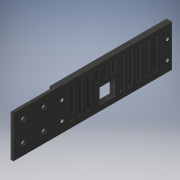
# Autodesk Inventor part: Base Left Front Panel
Saved by Autodesk Inventor 2019 (Build 230136000, 136)
## iProperties
Created: 2018-11-05
Part Number: Base Left Front Panel
Material: Generic
Document SubType Name: Modeling
Designer: Keith
Density: 1 g/cm^3
Appearance: Default
Author: Keith
## iProperties of the stored document Base Left Front Panel_3DPrint.ipt
Created: 2018-12-04
Part Number: Base Left Front Panel_3DPrint
Material: Generic
Document SubType Name: Modeling
Designer: Keith
Density: 1 g/cm^3
Appearance: Default
Author: Keith
Autodesk Inventor part; units mm, degrees
(part 1 of 2)
ref_plane "YZ Plane" through (0, 0, 0) normal (1, 0, 0) x (0, 1, 0)
sketch "Sketch1" plane through (0, 0, 0) normal (0, 1, 0) x (-1, 0, 0)
  line L0 (0, 0) -> (124, 0)
  line L1 (124, 0) -> (124, -124.7)
  line L2 (124, -124.7) -> (0, -124.7)
  line L3 (0, -124.7) -> (0, 0)
  line L4 (121.5, -2.5) -> (2.5, -2.5)
  line L5 (2.5, -2.5) -> (2.5, -122.2)
  line L6 (2.5, -122.2) -> (121.5, -122.2)
  line L7 (121.5, -122.2) -> (121.5, -2.5)
  line L8 (113, -2.5) -> (121.5, -2.5)
  line L9 (121.5, -2.5) -> (121.5, -11.25)
  line L10 (121.5, -11.25) -> (113, -11.25)
  line L11 (113, -11.25) -> (113, -2.5)
  line L12 (2.5, -11.25) -> (11, -11.25)
  line L13 (11, -11.25) -> (11, -2.5)
  line L14 (124, -124.7) -> (113, -124.7)
  line L15 (113, -124.7) -> (113, -112.7)
  line L16 (124, -112.7) -> (124, -124.7)
  line L17 (124, -112.7) -> (124, -104.2)
  line L18 (124, -104.2) -> (113, -104.2)
  line L19 (113, -104.2) -> (113, -112.7)
  line L20 (11, -124.7) -> (11, -112.7)
  line L21 (0, -104.2) -> (11, -104.2)
  line L22 (11, -104.2) -> (11, -112.7)
  line L23 (11, -11.25) -> (2.5, -11.25)
  line L24 (2.5, -11.25) -> (2.5, -2.5)
  line L25 (2.5, -2.5) -> (11, -2.5)
  line L26 (11, -2.5) -> (11, -11.25)
  line L27 (0, -104.2) -> (11, -104.2)
  line L28 (11, -104.2) -> (11, -124.7)
  line L29 (11, -124.7) -> (0, -124.7)
  line L30 (0, -124.7) -> (0, -104.2)
  dimension "d0" = 124
  dimension "d1" = 124.7
  dimension "d2" = 2.5
  dimension "d3" = 2.5
  dimension "d4" = 2.5
  dimension "d5" = 2.5
  dimension "d6" = 11.25
  dimension "d7" = 11
  dimension "d8" = 12
  dimension "d9" = 11
  dimension "d10" = 8.5
  dimension "d125" = 0
  dimension "d126" = 20.5
  constraints: 62 end point, 12 parallel, 6 horizontal, 6 perpendicular, 3 point on line
  measures "d0" distance of L1.end L2.end
  measures "d1" distance of L0.end L1.end
  measures "d2" distance between parallel lines of L1 L7
  measures "d3" distance between parallel lines of L0 L4
  measures "d4" distance between parallel lines of L3 L5
  measures "d5" distance between parallel lines of L2 L6
  measures "d6" distance between parallel lines of L0 L10
  measures "d7" distance between parallel lines of L1 L11
  measures "d8" distance of L14.end L15.end
  measures "d9" distance between parallel lines of L1 L15
  measures "d10" distance of L17.end L17.start
  measures "d125" distance between parallel lines of L2 L29
  measures "d126" distance between parallel lines of L2 L21
extrude "Extrusion1" add sketch "Sketch1" along normal blind 43 contours L0 L1 L18 L7 L4 L5 L21 L3 | L21 L5 L6 L20 L2 L3 | L1 L2 L15 L6 L7 L18 | L21 L22 L20 L6 L5 | L7 L6 L15 L19 L18 | L20 L6 L15 L2 | L5 L4 L13 L12 | L10 L11 L4 L7
sketch "Sketch2" plane through (0, 43, 0) normal (0, 1, 0) x (1, 0, 0)
  line L0 (-124, 124.7) -> (-124, 0) projected
  line L1 (-124, 0) -> (0, 0) projected
  line L2 (0, 0) -> (0, 124.7) projected
  line L3 (0, 124.7) -> (-124, 124.7) projected
  line L4 (-113, 122.2) -> (-113, 104.2) projected
  line L5 (-113, 122.2) -> (-11, 122.2) projected
  line L6 (-11, 104.2) -> (-11, 122.2) projected
  line L7 (-2.5, 104.2) -> (-11, 104.2) projected
  line L8 (-2.5, 104.2) -> (-2.5, 11.25) projected
  line L9 (-11, 11.25) -> (-2.5, 11.25) projected
  line L10 (-11, 2.5) -> (-11, 11.25) projected
  line L11 (-11, 2.5) -> (-113, 2.5) projected
  line L12 (-113, 2.5) -> (-113, 11.25) projected
  line L13 (-113, 11.25) -> (-121.5, 11.25) projected
  line L14 (-121.5, 11.25) -> (-121.5, 104.2) projected
  line L15 (-113, 104.2) -> (-121.5, 104.2) projected
  line L16 (-124, 124.7) -> (-124, 0) projected
  line L17 (0, 131.353) -> (-124, 131.353)
  line L18 (-124, 131.353) -> (-124, 119.353)
  line L19 (0, 119.353) -> (0, 131.353)
  line L20 (-11, 104.2) -> (-11, 122.2) projected
  line L21 (-113, 119.353) -> (-113, 122.2)
  line L22 (-113, 122.2) -> (-11, 122.2)
  line L23 (-11, 122.2) -> (-11, 119.353)
  line L24 (-124, 119.353) -> (-113, 119.353)
  line L25 (-11, 119.353) -> (0, 119.353)
  dimension "d13" = 12
  constraints: 16 end point, 3 equal length, 2 horizontal, 2 point on line, 1 perpendicular
  measures "d13" distance of L18.end L17.end
extrude "Extrusion2" cut sketch "Sketch2" against normal blind 11.4 contours L3 L2 L25 L6 L5 L4 L24 L0 | L18 L17 L19 L3
sketch "Sketch3" plane through (0, 31.6, 0) normal (0, 1, 0) x (1, 0, 0)
  line L0 (-124, 124.7) -> (0, 124.7) projected
  line L1 (-124, 124.7) -> (0, 124.7) projected
  line L2 (-124, 119.353) -> (-124, 124.7) projected
  line L3 (-113, 119.353) -> (-124, 119.353) projected
  line L4 (-113, 122.2) -> (-113, 119.353) projected
  line L5 (-11, 122.2) -> (-113, 122.2) projected
  line L6 (-11, 119.353) -> (-11, 122.2) projected
  line L7 (0, 119.353) -> (-11, 119.353) projected
  line L8 (0, 124.7) -> (0, 119.353) projected
  line L9 (-113, 122.2) -> (-11, 122.2)
  line L10 (-11, 122.2) -> (-11, 124.7)
  line L11 (-11, 124.7) -> (-113, 124.7)
  line L12 (-113, 124.7) -> (-113, 122.2)
  point P0 (0, 0)
  constraints: 8 end point, 2 parallel, 1 horizontal, 1 perpendicular, 1 point on line
extrude "Extrusion3" cut sketch "Sketch3" against normal through all contours L0 L10 L5 L12
sketch "Sketch4" plane through (0, 0, 0) normal (0, -1, 0) x (1, 0, 0)
  line L0 (-113, -104.2) -> (-113, -124.7) projected
  line L1 (-121.5, -104.2) -> (-113, -104.2) projected
  line L2 (-121.5, -104.2) -> (-121.5, -11.25) projected
  line L3 (-121.5, -11.25) -> (-113, -11.25) projected
  line L4 (-113, -11.25) -> (-113, -2.5) projected
  line L5 (-113, -2.5) -> (-11, -2.5) projected
  line L6 (-11, -11.25) -> (-11, -2.5) projected
  line L7 (-2.5, -11.25) -> (-11, -11.25) projected
  line L8 (-2.5, -11.25) -> (-2.5, -104.2) projected
  line L9 (-11, -104.2) -> (-2.5, -104.2) projected
  line L10 (-11, -104.2) -> (-11, -124.7) projected
  line L11 (0, -124.7) -> (-11, -124.7) projected
  line L12 (0, 0) -> (0, -124.7) projected
  line L13 (-124, 0) -> (0, 0) projected
  line L14 (-124, -124.7) -> (-124, 0) projected
  line L15 (0, -124.7) -> (-11, -124.7) projected
  line L16 (0, -124.7) -> (-124, -124.7)
  line L17 (-124, -124.7) -> (-124, 0)
  line L18 (-124, 0) -> (0, 0)
  line L19 (0, 0) -> (0, -124.7)
  line L20 (-113, -124.7) -> (-124, -124.7) projected
  constraints: 8 end point, 2 parallel, 1 horizontal, 1 perpendicular
extrude "Extrusion4" add sketch "Sketch4" against normal blind 2 contours L1 L2 L3 L4 L5 L6 L7 L8 L9 L10 L16 L0
sketch "Sketch5" plane through (-124, 0, -131.353) normal (-1, 0, 0) x (0, 0, 1)
  line L0 (12, 43) -> (12, 31.6) projected
  line L1 (12, 31.6) -> (6.653, 31.6) projected
  line L2 (6.653, 0) -> (6.653, 31.6) projected
  line L3 (131.353, 0) -> (131.353, 43) projected
  line L4 (12, 43) -> (131.353, 43) projected
  line L5 (66.653, 35) -> (119.903, 35)
  line L6 (119.903, 35) -> (119.903, 4)
  line L7 (119.903, 4) -> (66.653, 4)
  line L8 (66.653, 4) -> (66.653, 35)
  line L9 (6.653, 0) -> (131.353, 0) projected
  point P0 (131.353, 0)
  dimension "d21" = 31
  dimension "d129" = 113.25
  constraints: 8 end point, 2 parallel, 1 horizontal, 1 perpendicular
  measures "d21" distance of L5.end L6.end
  measures "d129" distance between parallel lines of L6 L2
extrude "Extrusion5" cut sketch "Sketch5" against normal blind 2.5 contours L5 L6 L7 L8
sketch "Sketch6" plane through (0, 43, 0) normal (0, 1, 0) x (1, 0, 0)
  line L0 (-113, 119.353) -> (-124, 119.353) projected
  line L1 (-124, 119.353) -> (-124, 0) projected
  line L2 (-124, 0) -> (0, 0) projected
  line L3 (0, 0) -> (0, 119.353) projected
  line L4 (0, 119.353) -> (-11, 119.353) projected
  line L5 (-11, 104.2) -> (-11, 119.353) projected
  line L6 (-2.5, 104.2) -> (-11, 104.2) projected
  line L7 (-2.5, 104.2) -> (-2.5, 11.25) projected
  line L8 (-11, 11.25) -> (-2.5, 11.25) projected
  line L9 (-11, 2.5) -> (-11, 11.25) projected
  line L10 (-11, 2.5) -> (-113, 2.5) projected
  line L11 (-113, 2.5) -> (-113, 11.25) projected
  line L12 (-113, 11.25) -> (-121.5, 11.25) projected
  line L13 (-121.5, 11.25) -> (-121.5, 104.2) projected
  line L14 (-113, 104.2) -> (-121.5, 104.2) projected
  line L15 (-113, 119.353) -> (-113, 104.2) projected
  line L16 (-11, 124.7) -> (-11, 104.2) projected
  line L17 (-11, 124.7) -> (-113, 124.7) projected
  line L18 (-113, 104.2) -> (-113, 124.7) projected
  line L19 (-121.5, 104.2) -> (-113, 104.2) projected
  line L20 (-121.5, 11.25) -> (-121.5, 104.2) projected
  line L21 (-113, 11.25) -> (-121.5, 11.25) projected
  line L22 (-113, 2.5) -> (-113, 11.25) projected
  line L23 (-11, 2.5) -> (-113, 2.5) projected
  line L24 (-11, 11.25) -> (-11, 2.5) projected
  line L25 (-2.5, 11.25) -> (-11, 11.25) projected
  line L26 (-2.5, 104.2) -> (-2.5, 11.25) projected
  line L27 (-11, 104.2) -> (-2.5, 104.2) projected
  line L28 (-11, 124.7) -> (-113, 124.7) projected
  line L29 (-62, 124.7) -> (-62, 28.7359)
  point P0 (-6.625, 6.875)
  point P1 (-6.625, 108.45)
  point P2 (-117.375, 6.875)
  point P3 (-117.375, 108.45)
  dimension "d27" = 4.375
  dimension "d28" = 4.375
  dimension "d29" = 4.25
  dimension "d30" = 4.375
  constraints: 2 end point, 2 symmetric about line, 1 midpoint, 1 vertical
  measures "d27" distance from line of L9 point (-6.625, 6.875)
  measures "d28" distance from line of L8 point (-6.625, 6.875)
  measures "d29" distance from line of L6 point (-6.625, 108.45)
  measures "d30" distance from line of L5 point (-6.625, 108.45)
hole "Hole1" at (-6.625, 43, -6.875) at (-6.625, 43, -108.45) at (-117.375, 43, -6.875) at (-117.375, 43, -108.45) direction (0, -1, 0) diameter 2.7 depth 12 tip angle 118
sketch "Sketch10" plane through (0, 0, 0) normal (1, 0, 0) x (0, 0, -1)
  line L0 (119.353, 31.6) -> (119.353, 43) projected
  line L1 (0, 43) -> (119.353, 43) projected
  line L2 (0, 0) -> (0, 43) projected
  line L3 (0, 0) -> (124.7, 0) projected
  line L4 (124.7, 31.6) -> (119.353, 31.6) projected
  line L5 (23.0532, 35.5) -> (27.0532, 35.5)
  line L6 (27.0532, 35.5) -> (27.0532, 5.5)
  line L7 (27.0532, 5.5) -> (23.0532, 5.5)
  line L8 (23.0532, 5.5) -> (23.0532, 35.5)
  line L9 (31.0532, 35.5) -> (35.0532, 35.5)
  line L10 (35.0532, 35.5) -> (35.0532, 5.5)
  line L11 (35.0532, 5.5) -> (31.0532, 5.5)
  line L12 (31.0532, 5.5) -> (31.0532, 35.5)
  line L13 (39.0532, 35.5) -> (43.0532, 35.5)
  line L14 (43.0532, 35.5) -> (43.0532, 5.5)
  line L15 (43.0532, 5.5) -> (39.0532, 5.5)
  line L16 (39.0532, 5.5) -> (39.0532, 35.5)
  line L17 (47.0532, 35.5) -> (51.0532, 35.5)
  line L18 (51.0532, 35.5) -> (51.0532, 5.5)
  line L19 (51.0532, 5.5) -> (47.0532, 5.5)
  line L20 (47.0532, 5.5) -> (47.0532, 35.5)
  line L21 (55.0532, 35.5) -> (59.0532, 35.5)
  line L22 (59.0532, 35.5) -> (59.0532, 5.5)
  line L23 (59.0532, 5.5) -> (55.0532, 5.5)
  line L24 (55.0532, 5.5) -> (55.0532, 35.5)
  line L25 (63.0532, 35.5) -> (67.0532, 35.5)
  line L26 (67.0532, 35.5) -> (67.0532, 5.5)
  line L27 (67.0532, 5.5) -> (63.0532, 5.5)
  line L28 (63.0532, 5.5) -> (63.0532, 35.5)
  line L29 (71.0532, 35.5) -> (75.0532, 35.5)
  line L30 (75.0532, 35.5) -> (75.0532, 5.5)
  line L31 (75.0532, 5.5) -> (71.0532, 5.5)
  line L32 (71.0532, 5.5) -> (71.0532, 35.5)
  line L33 (79.0532, 35.5) -> (83.0532, 35.5)
  line L34 (83.0532, 35.5) -> (83.0532, 5.5)
  line L35 (83.0532, 5.5) -> (79.0532, 5.5)
  line L36 (79.0532, 5.5) -> (79.0532, 35.5)
  line L37 (87.0532, 35.5) -> (91.0532, 35.5)
  line L38 (91.0532, 35.5) -> (91.0532, 5.5)
  line L39 (91.0532, 5.5) -> (87.0532, 5.5)
  line L40 (87.0532, 5.5) -> (87.0532, 35.5)
  line L41 (19.0532, 35.5) -> (15.0532, 35.5)
  line L42 (15.0532, 35.5) -> (15.0532, 5.5)
  line L43 (15.0532, 5.5) -> (19.0532, 5.5)
  line L44 (19.0532, 5.5) -> (19.0532, 35.5)
  line L45 (95.0532, 35.5) -> (99.0532, 35.5)
  line L46 (99.0532, 35.5) -> (99.0532, 5.5)
  line L47 (99.0532, 5.5) -> (95.0532, 5.5)
  line L48 (95.0532, 5.5) -> (95.0532, 35.5)
  line L49 (103.0532, 35.5) -> (107.0532, 35.5)
  line L50 (107.0532, 35.5) -> (107.0532, 5.5)
  line L51 (107.0532, 5.5) -> (103.0532, 5.5)
  line L52 (103.0532, 5.5) -> (103.0532, 35.5)
  line L53 (124.7, 0) -> (124.7, 31.6) projected
  dimension "d77" = 4
  dimension "d78" = 30
  dimension "d79" = 4
  dimension "d80" = 4
  dimension "d81" = 4
  dimension "d82" = 4
  dimension "d83" = 4
  dimension "d84" = 4
  dimension "d85" = 4
  dimension "d86" = 4
  dimension "d87" = 4
  dimension "d88" = 4
  dimension "d89" = 4
  dimension "d90" = 4
  dimension "d91" = 4
  dimension "d92" = 4
  dimension "d93" = 4
  dimension "d94" = 4
  dimension "d95" = 4
  dimension "d96" = 4
  dimension "d97" = 4
  dimension "d98" = 4
  dimension "d99" = 4
  dimension "d100" = 4
  dimension "d192" = 30
  dimension "d193" = 7.5
  dimension "d194" = 7.5
  constraints: 96 end point, 24 parallel, 20 point on line, 12 horizontal, 12 perpendicular
  measures "d77" distance of L6.end L7.end
  measures "d78" distance of L5.end L6.end
  measures "d79" distance of L10.end L11.end
  measures "d80" distance of L14.end L15.end
  measures "d81" distance of L18.end L19.end
  measures "d82" distance of L22.end L23.end
  measures "d83" distance of L26.end L27.end
  measures "d84" distance of L30.end L31.end
  measures "d85" distance of L34.end L35.end
  measures "d86" distance of L38.end L39.end
  measures "d87" distance of L43.end L42.end
  measures "d88" distance of L46.end L47.end
  measures "d89" distance of L50.end L51.end
  measures "d90" distance between parallel lines of L8 L44
  measures "d91" distance between parallel lines of L12 L6
  measures "d92" distance between parallel lines of L16 L10
  measures "d93" distance between parallel lines of L20 L14
  measures "d94" distance between parallel lines of L24 L18
  measures "d95" distance between parallel lines of L28 L22
  measures "d96" distance between parallel lines of L32 L26
  measures "d97" distance between parallel lines of L36 L30
  measures "d98" distance between parallel lines of L40 L34
  measures "d99" distance between parallel lines of L48 L38
  measures "d100" distance between parallel lines of L52 L46
  measures "d192" distance between parallel lines of L43 L41
  measures "d193" distance between parallel lines of L1 L41
  measures "d194" distance between parallel lines of L1 L5
extrude "Extrusion9" cut sketch "Sketch10" against normal through all contours L5 L6 L7 L8 | L9 L10 L11 L12 | L13 L14 L15 L16 | L17 L18 L19 L20 | L21 L22 L23 L24 | L25 L26 L27 L28 | L29 L30 L31 L32 | L33 L34 L35 L36 | L37 L38 L39 L40 | L44 L43 L42 L41 | L45 L46 L47 L48 | L49 L50 L51 L52
sketch "Sketch12" plane through (0, 31.6, 0) normal (0, 1, 0) x (1, 0, 0)
  line L0 (-113, 124.7) -> (-113, 119.353) projected
  line L1 (-124, 124.7) -> (-113, 124.7) projected
  line L2 (-124, 119.353) -> (-124, 124.7) projected
  line L3 (-113, 119.353) -> (-124, 119.353) projected
  line L4 (-11, 124.7) -> (-11, 119.353) projected
  line L5 (0, 119.353) -> (-11, 119.353) projected
  line L6 (0, 124.7) -> (0, 119.353) projected
  line L7 (-11, 124.7) -> (0, 124.7) projected
  line L8 (-7, 124.7) -> (-7, 126.2)
  line L9 (-4, 124.7) -> (-4, 126.2)
  line L10 (-7, 126.2) -> (-9.5, 126.2)
  line L11 (-4, 126.2) -> (-1.5, 126.2)
  line L12 (-1.5, 126.2) -> (-1.5, 127.2)
  line L13 (-9.5, 126.2) -> (-9.5, 127.2)
  line L14 (-9.5, 127.2) -> (-7, 129.7)
  line L15 (-9.5, 127.2) -> (-5.9645, 127.2) construction
  line L16 (-1.5, 127.2) -> (-4, 129.7)
  line L17 (-4, 129.7) -> (-7, 129.7)
  point P0 (0, 0)
  dimension "d105" = 1.5
  dimension "d106" = 1.5
  dimension "d107" = 4
  dimension "d108" = 4
  dimension "d109" = 2.5
  dimension "d110" = 2.5
  dimension "d111" = 1
  dimension "d112" = 1
  dimension "d113" = 45
  constraints: 20 end point, 4 horizontal, 3 vertical, 2 point on line, 1 equal length, 1 perpendicular
  measures "d105" distance of L8.start L8.end
  measures "d106" distance of L9.start L9.end
  measures "d107" distance between parallel lines of L4 L8
  measures "d108" distance between parallel lines of L6 L9
  measures "d109" distance of L8.end L10.end
  measures "d110" distance of L9.end L11.end
  measures "d111" distance of L11.end L12.end
  measures "d112" distance of L10.end L13.end
  measures "d113" angle of L15 L14
extrude "Extrusion11" add sketch "Sketch12" against normal up to surface (31.6 mm away) contours L8 L10 L13 L14 L17 L16 L12 L11 L9 L7
ref_plane "Work Plane1" through (-62, 31.6, -119.353) normal (1, 0, 0) x (0, 0, -1)
sketch "Sketch13" plane through (0, 0, 0) normal (1, 0, 0) x (0, 0, -1)
  line L0 (95.0532, 5.5) -> (95.0532, 35.5) projected
  line L1 (95.0532, 35.5) -> (99.0532, 35.5) projected
  line L2 (99.0532, 35.5) -> (99.0532, 5.5) projected
  line L3 (99.0532, 5.5) -> (95.0532, 5.5) projected
  line L4 (87.0532, 5.5) -> (87.0532, 35.5) projected
  line L5 (87.0532, 35.5) -> (91.0532, 35.5) projected
  line L6 (91.0532, 35.5) -> (91.0532, 5.5) projected
  line L7 (91.0532, 5.5) -> (87.0532, 5.5) projected
  line L8 (71.0532, 5.5) -> (71.0532, 35.5) projected
  line L9 (71.0532, 35.5) -> (75.0532, 35.5) projected
  line L10 (75.0532, 35.5) -> (75.0532, 5.5) projected
  line L11 (75.0532, 5.5) -> (71.0532, 5.5) projected
  line L12 (55.0532, 5.5) -> (55.0532, 35.5) projected
  line L13 (55.0532, 35.5) -> (59.0532, 35.5) projected
  line L14 (59.0532, 35.5) -> (59.0532, 5.5) projected
  line L15 (59.0532, 5.5) -> (55.0532, 5.5) projected
  line L16 (39.0532, 5.5) -> (39.0532, 35.5) projected
  line L17 (39.0532, 35.5) -> (43.0532, 35.5) projected
  line L18 (43.0532, 35.5) -> (43.0532, 5.5) projected
  line L19 (43.0532, 5.5) -> (39.0532, 5.5) projected
  line L20 (23.0532, 5.5) -> (23.0532, 35.5) projected
  line L21 (23.0532, 35.5) -> (27.0532, 35.5) projected
  line L22 (27.0532, 35.5) -> (27.0532, 5.5) projected
  line L23 (27.0532, 5.5) -> (23.0532, 5.5) projected
  line L24 (31.0532, 5.5) -> (31.0532, 35.5) projected
  line L25 (31.0532, 35.5) -> (35.0532, 35.5) projected
  line L26 (35.0532, 35.5) -> (35.0532, 5.5) projected
  line L27 (35.0532, 5.5) -> (31.0532, 5.5) projected
  line L28 (47.0532, 5.5) -> (47.0532, 35.5) projected
  line L29 (47.0532, 35.5) -> (51.0532, 35.5) projected
  line L30 (51.0532, 35.5) -> (51.0532, 5.5) projected
  line L31 (51.0532, 5.5) -> (47.0532, 5.5) projected
  line L32 (63.0532, 5.5) -> (63.0532, 35.5) projected
  line L33 (63.0532, 35.5) -> (67.0532, 35.5) projected
  line L34 (67.0532, 35.5) -> (67.0532, 5.5) projected
  line L35 (67.0532, 5.5) -> (63.0532, 5.5) projected
  line L36 (79.0532, 5.5) -> (79.0532, 35.5) projected
  line L37 (79.0532, 35.5) -> (83.0532, 35.5) projected
  line L38 (83.0532, 35.5) -> (83.0532, 5.5) projected
  line L39 (83.0532, 5.5) -> (79.0532, 5.5) projected
  line L40 (15.0532, 5.5) -> (15.0532, 35.5) projected
  line L41 (15.0532, 35.5) -> (19.0532, 35.5) projected
  line L42 (19.0532, 35.5) -> (19.0532, 5.5) projected
  line L43 (19.0532, 5.5) -> (15.0532, 5.5) projected
  line L44 (103.0532, 5.5) -> (103.0532, 35.5) projected
  line L45 (103.0532, 35.5) -> (107.0532, 35.5) projected
  line L46 (107.0532, 35.5) -> (107.0532, 5.5) projected
  line L47 (107.0532, 5.5) -> (103.0532, 5.5) projected
  line L48 (119.353, 31.6) -> (119.353, 43) projected
  line L49 (0, 43) -> (119.353, 43) projected
  line L50 (0, 0) -> (0, 43) projected
  line L51 (0, 0) -> (124.7, 0) projected
  line L52 (124.7, 31.6) -> (119.353, 31.6) projected
  line L53 (66, 17.8) -> (82, 17.8)
  line L54 (82, 17.8) -> (82, 5)
  line L55 (82, 5) -> (66, 5)
  line L56 (66, 5) -> (66, 17.8)
  line L57 (124.7, 0) -> (124.7, 31.6) projected
  dimension "d116" = 16
  dimension "d117" = 12.8
  dimension "d119" = 5
  constraints: 8 end point, 2 parallel, 1 horizontal, 1 perpendicular
  measures "d116" distance of L53.start L53.end
  measures "d117" distance between parallel lines of L55 L53
  measures "d119" distance between parallel lines of L51 L55
extrude "Extrusion12" cut sketch "Sketch13" against normal blind 2.5 contours L11 L10 L53 L36 L39 L54 L55 L56 L35 L34 L8 | L8 L53 L10 L11 | L34 L35 L56 L53 | L53 L54 L39 L36
sketch "Sketch14" plane through (0, 0, 0) normal (1, 0, 0) x (0, 0, -1)
  line L0 (66, 5) -> (66, 5.5) projected
  line L1 (66, 5.5) -> (63.0532, 5.5) projected
  line L2 (63.0532, 5.5) -> (63.0532, 35.5) projected
  line L3 (63.0532, 35.5) -> (67.0532, 35.5) projected
  line L4 (67.0532, 35.5) -> (67.0532, 17.8) projected
  line L5 (67.0532, 17.8) -> (71.0532, 17.8) projected
  line L6 (71.0532, 17.8) -> (71.0532, 35.5) projected
  line L7 (71.0532, 35.5) -> (75.0532, 35.5) projected
  line L8 (75.0532, 35.5) -> (75.0532, 17.8) projected
  line L9 (75.0532, 17.8) -> (79.0532, 17.8) projected
  line L10 (79.0532, 17.8) -> (79.0532, 35.5) projected
  line L11 (79.0532, 35.5) -> (83.0532, 35.5) projected
  line L12 (83.0532, 35.5) -> (83.0532, 5.5) projected
  line L13 (83.0532, 5.5) -> (82, 5.5) projected
  line L14 (82, 5.5) -> (82, 5) projected
  line L15 (82, 5) -> (66, 5) projected
  line L16 (95.0532, 5.5) -> (95.0532, 35.5) projected
  line L17 (95.0532, 35.5) -> (99.0532, 35.5) projected
  line L18 (99.0532, 35.5) -> (99.0532, 5.5) projected
  line L19 (99.0532, 5.5) -> (95.0532, 5.5) projected
  line L20 (87.0532, 5.5) -> (87.0532, 35.5) projected
  line L21 (87.0532, 35.5) -> (91.0532, 35.5) projected
  line L22 (91.0532, 35.5) -> (91.0532, 5.5) projected
  line L23 (91.0532, 5.5) -> (87.0532, 5.5) projected
  line L24 (55.0532, 5.5) -> (55.0532, 35.5) projected
  line L25 (55.0532, 35.5) -> (59.0532, 35.5) projected
  line L26 (59.0532, 35.5) -> (59.0532, 5.5) projected
  line L27 (59.0532, 5.5) -> (55.0532, 5.5) projected
  line L28 (39.0532, 5.5) -> (39.0532, 35.5) projected
  line L29 (39.0532, 35.5) -> (43.0532, 35.5) projected
  line L30 (43.0532, 35.5) -> (43.0532, 5.5) projected
  line L31 (43.0532, 5.5) -> (39.0532, 5.5) projected
  line L32 (23.0532, 5.5) -> (23.0532, 35.5) projected
  line L33 (23.0532, 35.5) -> (27.0532, 35.5) projected
  line L34 (27.0532, 35.5) -> (27.0532, 5.5) projected
  line L35 (27.0532, 5.5) -> (23.0532, 5.5) projected
  line L36 (31.0532, 5.5) -> (31.0532, 35.5) projected
  line L37 (31.0532, 35.5) -> (35.0532, 35.5) projected
  line L38 (35.0532, 35.5) -> (35.0532, 5.5) projected
  line L39 (35.0532, 5.5) -> (31.0532, 5.5) projected
  line L40 (47.0532, 5.5) -> (47.0532, 35.5) projected
  line L41 (47.0532, 35.5) -> (51.0532, 35.5) projected
  line L42 (51.0532, 35.5) -> (51.0532, 5.5) projected
  line L43 (51.0532, 5.5) -> (47.0532, 5.5) projected
  line L44 (15.0532, 5.5) -> (15.0532, 35.5) projected
  line L45 (15.0532, 35.5) -> (19.0532, 35.5) projected
  line L46 (19.0532, 35.5) -> (19.0532, 5.5) projected
  line L47 (19.0532, 5.5) -> (15.0532, 5.5) projected
  line L48 (103.0532, 5.5) -> (103.0532, 35.5) projected
  line L49 (103.0532, 35.5) -> (107.0532, 35.5) projected
  line L50 (107.0532, 35.5) -> (107.0532, 5.5) projected
  line L51 (107.0532, 5.5) -> (103.0532, 5.5) projected
  line L52 (119.353, 31.6) -> (119.353, 43) projected
  line L53 (0, 43) -> (119.353, 43) projected
  line L54 (0, 0) -> (0, 43) projected
  line L55 (0, 0) -> (124.7, 0) projected
  line L56 (124.7, 31.6) -> (119.353, 31.6) projected
  line L57 (63.0532, 35.5) -> (63.0532, 5.5) projected
  line L58 (67.0532, 17.8) -> (63.0532, 17.8)
  line L59 (63.0532, 17.8) -> (63.0532, 21.8)
  line L60 (63.0532, 21.8) -> (67.0532, 21.8)
  line L61 (67.0532, 21.8) -> (67.0532, 17.8)
  line L62 (79.0532, 17.8) -> (83.0532, 17.8)
  line L63 (83.0532, 17.8) -> (83.0532, 21.8)
  line L64 (83.0532, 21.8) -> (79.0532, 21.8)
  line L65 (79.0532, 21.8) -> (79.0532, 17.8)
  line L66 (83.0532, 5.5) -> (79.0532, 5.5) projected
  line L67 (83.0532, 5.5) -> (82, 5.5)
  line L68 (82, 5.5) -> (82, 17.8)
  line L69 (82, 17.8) -> (83.0532, 17.8)
  line L70 (83.0532, 17.8) -> (83.0532, 5.5)
  line L71 (66, 5.5) -> (63.0532, 5.5)
  line L72 (63.0532, 5.5) -> (63.0532, 17.9857)
  line L73 (63.0532, 17.9857) -> (66, 17.9857)
  line L74 (66, 17.9857) -> (66, 5.5)
  line L75 (71.0532, 35.5) -> (71.0532, 17.8) projected
  line L76 (75.0532, 17.8) -> (71.0532, 17.8)
  line L77 (71.0532, 17.8) -> (71.0532, 21.8)
  line L78 (71.0532, 21.8) -> (75.0532, 21.8)
  line L79 (75.0532, 21.8) -> (75.0532, 17.8)
  line L80 (124.7, 0) -> (124.7, 31.6) projected
  dimension "d122" = 4
  constraints: 40 end point, 10 parallel, 6 point on line, 5 horizontal, 5 perpendicular
  measures "d122" distance of L58.end L59.end
extrude "Extrusion13" add sketch "Sketch14" against normal blind 2.5 contours L1 L2 L58 L74 | L74 L73 L2 L60 L4 L58 | L58 L2 L73 L74 | L68 L62 L12 L13 | L62 L10 L64 L12 | L6 L78 L8 L76
mirror "Mirror2" about plane through (-62, 31.6, -119.353) normal (1, 0, 0) of "Extrusion11"
sketch "Sketch15" plane through (-124, 0, -124.7) normal (-1, 0, 0) x (0, 0, 1)
  line L0 (58.7, 5) -> (42.7, 5) projected
  line L1 (69.6468, 35.5) -> (69.6468, 35) projected
  line L2 (69.6468, 35) -> (73.6468, 35) projected
  line L3 (73.6468, 35) -> (73.6468, 35.5) projected
  line L4 (73.6468, 35.5) -> (77.6468, 35.5) projected
  line L5 (77.6468, 35.5) -> (77.6468, 35) projected
  line L6 (77.6468, 35) -> (81.6468, 35) projected
  line L7 (81.6468, 35) -> (81.6468, 35.5) projected
  line L8 (81.6468, 35.5) -> (85.6468, 35.5) projected
  line L9 (85.6468, 35.5) -> (85.6468, 35) projected
  line L10 (85.6468, 35) -> (89.6468, 35) projected
  line L11 (89.6468, 35) -> (89.6468, 35.5) projected
  line L12 (89.6468, 35.5) -> (93.6468, 35.5) projected
  line L13 (93.6468, 35.5) -> (93.6468, 35) projected
  line L14 (93.6468, 35) -> (97.6468, 35) projected
  line L15 (97.6468, 35) -> (97.6468, 35.5) projected
  line L16 (97.6468, 35.5) -> (101.6468, 35.5) projected
  line L17 (101.6468, 35.5) -> (101.6468, 35) projected
  line L18 (101.6468, 35) -> (105.6468, 35) projected
  line L19 (105.6468, 35) -> (105.6468, 35.5) projected
  line L20 (105.6468, 35.5) -> (109.6468, 35.5) projected
  line L21 (109.6468, 35.5) -> (109.6468, 35) projected
  line L22 (109.6468, 35) -> (113.25, 35) projected
  line L23 (113.25, 35) -> (113.25, 4) projected
  line L24 (113.25, 4) -> (60, 4) projected
  line L25 (60, 4) -> (60, 5.5) projected
  line L26 (60, 5.5) -> (57.6468, 5.5) projected
  line L27 (57.6468, 5.5) -> (57.6468, 35.5) projected
  line L28 (57.6468, 35.5) -> (61.6468, 35.5) projected
  line L29 (61.6468, 35.5) -> (61.6468, 35) projected
  line L30 (61.6468, 35) -> (65.6468, 35) projected
  line L31 (65.6468, 35) -> (65.6468, 35.5) projected
  line L32 (65.6468, 35.5) -> (69.6468, 35.5) projected
  line L33 (29.6468, 35.5) -> (29.6468, 5.5) projected
  line L34 (29.6468, 5.5) -> (25.6468, 5.5) projected
  line L35 (25.6468, 5.5) -> (25.6468, 35.5) projected
  line L36 (25.6468, 35.5) -> (29.6468, 35.5) projected
  line L37 (37.6468, 35.5) -> (37.6468, 5.5) projected
  line L38 (37.6468, 5.5) -> (33.6468, 5.5) projected
  line L39 (33.6468, 5.5) -> (33.6468, 35.5) projected
  line L40 (33.6468, 35.5) -> (37.6468, 35.5) projected
  line L41 (53.6468, 35.5) -> (53.6468, 5.5) projected
  line L42 (53.6468, 5.5) -> (49.6468, 5.5) projected
  line L43 (49.6468, 5.5) -> (49.6468, 35.5) projected
  line L44 (49.6468, 35.5) -> (53.6468, 35.5) projected
  line L45 (45.6468, 35.5) -> (45.6468, 5.5) projected
  line L46 (45.6468, 5.5) -> (41.6468, 5.5) projected
  line L47 (41.6468, 5.5) -> (41.6468, 35.5) projected
  line L48 (41.6468, 35.5) -> (45.6468, 35.5) projected
  line L49 (21.6468, 35.5) -> (21.6468, 5.5) projected
  line L50 (21.6468, 5.5) -> (17.6468, 5.5) projected
  line L51 (17.6468, 5.5) -> (17.6468, 35.5) projected
  line L52 (17.6468, 35.5) -> (21.6468, 35.5) projected
  line L53 (5.347, 43) -> (5.347, 31.6) projected
  line L54 (5.347, 31.6) -> (0, 31.6) projected
  line L55 (0, 0) -> (0, 31.6) projected
  line L56 (0, 0) -> (124.7, 0) projected
  line L57 (124.7, 0) -> (124.7, 43) projected
  line L58 (5.347, 43) -> (124.7, 43) projected
  line L59 (57.6468, 35.5) -> (57.6468, 5.5) projected
  line L60 (60, 5.5) -> (57.6468, 5.5)
  line L61 (57.6468, 5.5) -> (57.6468, 35.5)
  line L62 (57.6468, 35.5) -> (60, 35.5)
  line L63 (60, 35.5) -> (60, 5.5)
  line L64 (60, 32.5785) -> (116.515, 32.5785)
  line L65 (116.515, 32.5785) -> (116.515, 35.5)
  line L66 (116.515, 35.5) -> (60, 35.5)
  line L67 (60, 35.5) -> (60, 32.5785)
  point P0 (124.7, 0)
  constraints: 16 end point, 4 parallel, 2 horizontal, 2 perpendicular, 2 point on line
extrude "Extrusion14" add sketch "Sketch15" against normal blind 2.5 contours L66 L3 L2 L1 | L1 L2 L3 L4 L5 L6 L7 L8 L9 L10 L11 L12 L13 L14 L15 L16 L17 L18 L19 L20 L21 L22 L23 L64 L63 L28 L29 L30 L31 L32 | L31 L30 L29 L66 | L66 L7 L6 L5 | L63 L26 L27 L28 | L66 L11 L10 L9 | L23 L22 L21 L66 L65 L64 | L66 L15 L14 L13 | L66 L19 L18 L17
sketch "Sketch16" plane through (-124, 4, -11.45) normal (0, 0, -1) x (-1, 0, 0)
  line L0 (0, 28.5785) -> (0, 0) projected
  line L1 (-2.5, 0) -> (-2.5, 28.5785) projected
  line L2 (0, 0) -> (-2.5, 0) projected
  line L3 (0, 28.5785) -> (-2.5, 28.5785) projected
  point P0 (-124, -4)
extrude "Extrusion15" cut sketch "Sketch16" against normal up to surface (0.2 mm away)
sketch "Sketch17" plane through (0, 0, 0) normal (1, 0, 0) x (0, 0, -1)
  line L0 (79.0532, 21.8) -> (79.0532, 35.5) projected
  line L1 (79.0532, 35.5) -> (83.0532, 35.5) projected
  line L2 (83.0532, 35.5) -> (83.0532, 21.8) projected
  line L3 (83.0532, 21.8) -> (79.0532, 21.8) projected
  line L4 (66, 17.8) -> (82, 17.8) projected
  line L5 (82, 17.8) -> (82, 5) projected
  line L6 (82, 5) -> (66, 5) projected
  line L7 (66, 5) -> (66, 17.8) projected
  line L8 (63.0532, 21.8) -> (63.0532, 35.5) projected
  line L9 (63.0532, 35.5) -> (67.0532, 35.5) projected
  line L10 (67.0532, 35.5) -> (67.0532, 21.8) projected
  line L11 (67.0532, 21.8) -> (63.0532, 21.8) projected
  line L12 (75.0532, 21.8) -> (71.0532, 21.8) projected
  line L13 (71.0532, 21.8) -> (71.0532, 35.5) projected
  line L14 (71.0532, 35.5) -> (75.0532, 35.5) projected
  line L15 (75.0532, 35.5) -> (75.0532, 21.8) projected
  line L16 (95.0532, 5.5) -> (95.0532, 35.5) projected
  line L17 (95.0532, 35.5) -> (99.0532, 35.5) projected
  line L18 (99.0532, 35.5) -> (99.0532, 5.5) projected
  line L19 (99.0532, 5.5) -> (95.0532, 5.5) projected
  line L20 (87.0532, 5.5) -> (87.0532, 35.5) projected
  line L21 (87.0532, 35.5) -> (91.0532, 35.5) projected
  line L22 (91.0532, 35.5) -> (91.0532, 5.5) projected
  line L23 (91.0532, 5.5) -> (87.0532, 5.5) projected
  line L24 (55.0532, 5.5) -> (55.0532, 35.5) projected
  line L25 (55.0532, 35.5) -> (59.0532, 35.5) projected
  line L26 (59.0532, 35.5) -> (59.0532, 5.5) projected
  line L27 (59.0532, 5.5) -> (55.0532, 5.5) projected
  line L28 (39.0532, 5.5) -> (39.0532, 35.5) projected
  line L29 (39.0532, 35.5) -> (43.0532, 35.5) projected
  line L30 (43.0532, 35.5) -> (43.0532, 5.5) projected
  line L31 (43.0532, 5.5) -> (39.0532, 5.5) projected
  line L32 (23.0532, 5.5) -> (23.0532, 35.5) projected
  line L33 (23.0532, 35.5) -> (27.0532, 35.5) projected
  line L34 (27.0532, 35.5) -> (27.0532, 5.5) projected
  line L35 (27.0532, 5.5) -> (23.0532, 5.5) projected
  line L36 (31.0532, 5.5) -> (31.0532, 35.5) projected
  line L37 (31.0532, 35.5) -> (35.0532, 35.5) projected
  line L38 (35.0532, 35.5) -> (35.0532, 5.5) projected
  line L39 (35.0532, 5.5) -> (31.0532, 5.5) projected
  line L40 (47.0532, 5.5) -> (47.0532, 35.5) projected
  line L41 (47.0532, 35.5) -> (51.0532, 35.5) projected
  line L42 (51.0532, 35.5) -> (51.0532, 5.5) projected
  line L43 (51.0532, 5.5) -> (47.0532, 5.5) projected
  line L44 (15.0532, 5.5) -> (15.0532, 35.5) projected
  line L45 (15.0532, 35.5) -> (19.0532, 35.5) projected
  line L46 (19.0532, 35.5) -> (19.0532, 5.5) projected
  line L47 (19.0532, 5.5) -> (15.0532, 5.5) projected
  line L48 (103.0532, 5.5) -> (103.0532, 35.5) projected
  line L49 (103.0532, 35.5) -> (107.0532, 35.5) projected
  line L50 (107.0532, 35.5) -> (107.0532, 5.5) projected
  line L51 (107.0532, 5.5) -> (103.0532, 5.5) projected
  line L52 (119.353, 31.6) -> (119.353, 43) projected
  line L53 (0, 43) -> (119.353, 43) projected
  line L54 (0, 0) -> (0, 43) projected
  line L55 (0, 0) -> (124.7, 0) projected
  line L56 (124.7, 0) -> (124.7, 31.6) projected
  line L57 (124.7, 31.6) -> (119.353, 31.6) projected
  line L58 (135.3554, 31.6) -> (124.7, 31.6)
  line L59 (135.3554, 31.6) -> (124.7, 31.6)
  line L60 (124.7, 31.6) -> (124.7, 30.6)
  line L61 (124.7, 30.6) -> (135.3554, 30.6)
  line L62 (135.3554, 30.6) -> (135.3554, 31.6)
  line L63 (135.3554, 31.6) -> (119.353, 31.6)
  line L64 (119.353, 31.6) -> (119.353, 30.6)
  line L65 (119.353, 30.6) -> (135.3554, 30.6)
  line L66 (135.3554, 30.6) -> (135.3554, 31.6)
  dimension "d134" = 1
  constraints: 18 end point, 4 parallel, 2 horizontal, 2 perpendicular
  measures "d134" distance of L60.end L59.end
extrude "Extrusion16" cut sketch "Sketch17" against normal through all contours L57 L56 L65 L64 | L58 L62 L61 L56
sketch "Sketch18" plane through (0, 43, 0) normal (0, 1, 0) x (1, 0, 0)
  circle A0 centre (-117.375, 6.875) radius 1.35 projected
  circle A1 centre (-6.625, 6.875) radius 1.35 projected
  circle A2 centre (-6.625, 108.45) radius 1.35 projected
  circle A3 centre (-117.375, 108.45) radius 1.35 projected
  line L0 (-113, 119.353) -> (-124, 119.353) projected
  line L1 (-124, 119.353) -> (-124, 0) projected
  line L2 (-124, 0) -> (0, 0) projected
  line L3 (0, 0) -> (0, 119.353) projected
  line L4 (0, 119.353) -> (-11, 119.353) projected
  line L5 (-11, 104.2) -> (-11, 119.353) projected
  line L6 (-2.5, 104.2) -> (-11, 104.2) projected
  line L7 (-2.5, 104.2) -> (-2.5, 11.25) projected
  line L8 (-11, 11.25) -> (-2.5, 11.25) projected
  line L9 (-11, 2.5) -> (-11, 11.25) projected
  line L10 (-11, 2.5) -> (-113, 2.5) projected
  line L11 (-113, 2.5) -> (-113, 11.25) projected
  line L12 (-113, 11.25) -> (-121.5, 11.25) projected
  line L13 (-121.5, 11.25) -> (-121.5, 104.2) projected
  line L14 (-113, 104.2) -> (-121.5, 104.2) projected
  line L15 (-113, 119.353) -> (-113, 104.2) projected
extrude "Extrusion17" cut sketch "Sketch18" along normal blind 3
sketch "Sketch19" plane through (0, 43, 0) normal (0, 1, 0) x (1, 0, 0)
  circle A0 centre (-117.375, 6.875) radius 1.35 projected
  circle A1 centre (-6.625, 6.875) radius 1.35 projected
  circle A2 centre (-6.625, 108.45) radius 1.35 projected
  circle A3 centre (-117.375, 108.45) radius 1.35 projected
  line L0 (-113, 119.353) -> (-124, 119.353) projected
  line L1 (-124, 119.353) -> (-124, 0) projected
  line L2 (-124, 0) -> (0, 0) projected
  line L3 (0, 0) -> (0, 119.353) projected
  line L4 (0, 119.353) -> (-11, 119.353) projected
  line L5 (-11, 104.2) -> (-11, 119.353) projected
  line L6 (-2.5, 104.2) -> (-11, 104.2) projected
  line L7 (-2.5, 104.2) -> (-2.5, 11.25) projected
  line L8 (-11, 11.25) -> (-2.5, 11.25) projected
  line L9 (-11, 2.5) -> (-11, 11.25) projected
  line L10 (-11, 2.5) -> (-113, 2.5) projected
  line L11 (-113, 2.5) -> (-113, 11.25) projected
  line L12 (-113, 11.25) -> (-121.5, 11.25) projected
  line L13 (-121.5, 11.25) -> (-121.5, 104.2) projected
  line L14 (-113, 104.2) -> (-121.5, 104.2) projected
  line L15 (-113, 119.353) -> (-113, 104.2) projected
extrude "Extrusion18" cut sketch "Sketch19" against normal blind 3
sketch "Sketch21" plane through (0, 40, 0) normal (0, 1, 0) x (1, 0, 0)
  circle A0 centre (-117.375, 108.45) radius 1.35 projected
  circle A1 centre (-6.625, 108.45) radius 1.35 projected
  circle A2 centre (-6.625, 6.875) radius 1.35 projected
  circle A3 centre (-117.375, 6.875) radius 1.35 projected
  line L0 (-124, 119.353) -> (-113, 119.353) projected
  line L1 (-124, 0) -> (-124, 119.353) projected
  line L2 (0, 0) -> (-124, 0) projected
  line L3 (0, 119.353) -> (0, 0) projected
  line L4 (-11, 119.353) -> (0, 119.353) projected
  line L5 (-11, 104.2) -> (-11, 119.353) projected
  line L6 (-2.5, 104.2) -> (-11, 104.2) projected
  line L7 (-2.5, 11.25) -> (-2.5, 104.2) projected
  line L8 (-11, 11.25) -> (-2.5, 11.25) projected
  line L9 (-11, 2.5) -> (-11, 11.25) projected
  line L10 (-113, 2.5) -> (-11, 2.5) projected
  line L11 (-113, 11.25) -> (-113, 2.5) projected
  line L12 (-121.5, 11.25) -> (-113, 11.25) projected
  line L13 (-121.5, 104.2) -> (-121.5, 11.25) projected
  line L14 (-113, 104.2) -> (-121.5, 104.2) projected
  line L15 (-113, 119.353) -> (-113, 104.2) projected
  line L16 (-113, 119.353) -> (-124, 119.353)
  line L17 (-124, 119.353) -> (-124, 112.7)
  line L18 (-124, 112.7) -> (-113, 112.7)
  line L19 (-113, 112.7) -> (-113, 119.353)
  line L20 (-11, 119.353) -> (0, 119.353) projected
  line L21 (0, 119.353) -> (-11, 119.353)
  line L22 (-11, 119.353) -> (-11, 112.7)
  line L23 (-11, 112.7) -> (0, 112.7)
  line L24 (0, 112.7) -> (0, 119.353)
  line L25 (-11, 124.7) -> (-11, 104.2) projected
  line L26 (-11, 124.7) -> (-113, 124.7) projected
  line L27 (-113, 104.2) -> (-113, 124.7) projected
  line L28 (-121.5, 104.2) -> (-113, 104.2) projected
  line L29 (-121.5, 11.25) -> (-121.5, 104.2) projected
  line L30 (-113, 11.25) -> (-121.5, 11.25) projected
  line L31 (-113, 2.5) -> (-113, 11.25) projected
  line L32 (-11, 2.5) -> (-113, 2.5) projected
  line L33 (-11, 11.25) -> (-11, 2.5) projected
  line L34 (-2.5, 11.25) -> (-11, 11.25) projected
  line L35 (-2.5, 104.2) -> (-2.5, 11.25) projected
  line L36 (-11, 104.2) -> (-2.5, 104.2) projected
  dimension "d157" = 12
  constraints: 16 end point, 4 parallel, 3 point on line, 2 horizontal, 2 perpendicular
  measures "d157" distance between parallel lines of L26 L23
extrude "Extrusion20" cut sketch "Sketch21" against normal up to surface (9.4 mm away) contours L0 L15 L18 L1 | L4 L3 L23 L5
sketch "Sketch22" plane through (-113, 2, -104.2) normal (1, 0, 0) x (0, 0, -1)
  line L0 (20.5, 28.6) -> (8.5, 28.6) projected
  line L1 (8.5, 28.6) -> (8.5, 38) projected
  line L2 (8.5, 38) -> (0, 38) projected
  line L3 (0, 33.5) -> (0, 38) projected
  line L4 (0, 33.5) -> (2.8532, 33.5) projected
  line L5 (2.8532, 33.5) -> (2.8532, 3.5) projected
  line L6 (2.8532, 3.5) -> (0, 3.5) projected
  line L7 (0, 0) -> (0, 3.5) projected
  line L8 (0, 0) -> (20.5, 0) projected
  line L9 (20.5, 28.6) -> (20.5, 0) projected
  line L10 (0, 38) -> (-92.95, 38) projected
  line L11 (-92.95, 0) -> (-92.95, 2) projected
  line L12 (-39.5, 30.5785) -> (-39.5, 2) projected
  line L13 (-39.5, 2) -> (-92.95, 2) projected
  line L14 (-92.95, 30.5785) -> (-92.95, 38) projected
  line L15 (-92.95, 0) -> (0, 0) projected
  line L16 (0, 3.5) -> (0, 0) projected
  line L17 (0, 3.5) -> (-1.1468, 3.5) projected
  line L18 (-1.1468, 3.5) -> (-1.1468, 33.5) projected
  line L19 (-1.1468, 33.5) -> (0, 33.5) projected
  line L20 (0, 38) -> (0, 33.5) projected
  line L21 (-9.1468, 3.5) -> (-9.1468, 33.5) projected
  line L22 (-9.1468, 33.5) -> (-5.1468, 33.5) projected
  line L23 (-5.1468, 33.5) -> (-5.1468, 3.5) projected
  line L24 (-5.1468, 3.5) -> (-9.1468, 3.5) projected
  line L25 (-17.1468, 3.5) -> (-17.1468, 33.5) projected
  line L26 (-17.1468, 33.5) -> (-13.1468, 33.5) projected
  line L27 (-13.1468, 33.5) -> (-13.1468, 3.5) projected
  line L28 (-13.1468, 3.5) -> (-17.1468, 3.5) projected
  line L29 (-33.1468, 3.5) -> (-33.1468, 33.5) projected
  line L30 (-33.1468, 33.5) -> (-29.1468, 33.5) projected
  line L31 (-29.1468, 33.5) -> (-29.1468, 3.5) projected
  line L32 (-29.1468, 3.5) -> (-33.1468, 3.5) projected
  line L33 (-25.1468, 3.5) -> (-25.1468, 33.5) projected
  line L34 (-25.1468, 33.5) -> (-21.1468, 33.5) projected
  line L35 (-21.1468, 33.5) -> (-21.1468, 3.5) projected
  line L36 (-21.1468, 3.5) -> (-25.1468, 3.5) projected
  line L37 (2.8532, 33.5) -> (0, 33.5)
  line L38 (0, 33.5) -> (0, 3.5)
  line L39 (0, 3.5) -> (2.8532, 3.5)
  line L40 (2.8532, 3.5) -> (2.8532, 33.5)
  line L41 (-92.95, 30.5785) -> (-39.5, 30.5785) projected
  point P0 (-104.2, -2)
  constraints: 8 end point, 2 parallel, 1 horizontal, 1 perpendicular
extrude "Extrusion21" add sketch "Sketch22" against normal up to surface (11 mm away) contours L38 L4 L5 L6
sketch "Sketch23" plane through (-124, 0, -124.7) normal (-1, 0, 0) x (0, 0, 1)
  line L0 (12, 30.6) -> (0, 30.6) projected
  line L1 (0, 0) -> (0, 30.6) projected
  line L2 (0, 0) -> (124.7, 0) projected
  line L3 (124.7, 0) -> (124.7, 40) projected
  line L4 (124.7, 40) -> (12, 40) projected
  line L5 (12, 40) -> (12, 30.6) projected
  line L6 (29.6468, 35.5) -> (29.6468, 5.5) projected
  line L7 (29.6468, 5.5) -> (25.6468, 5.5) projected
  line L8 (25.6468, 5.5) -> (25.6468, 35.5) projected
  line L9 (25.6468, 35.5) -> (29.6468, 35.5) projected
  line L10 (37.6468, 35.5) -> (37.6468, 5.5) projected
  line L11 (37.6468, 5.5) -> (33.6468, 5.5) projected
  line L12 (33.6468, 5.5) -> (33.6468, 35.5) projected
  line L13 (33.6468, 35.5) -> (37.6468, 35.5) projected
  line L14 (53.6468, 35.5) -> (53.6468, 5.5) projected
  line L15 (53.6468, 5.5) -> (49.6468, 5.5) projected
  line L16 (49.6468, 5.5) -> (49.6468, 35.5) projected
  line L17 (49.6468, 35.5) -> (53.6468, 35.5) projected
  line L18 (45.6468, 35.5) -> (45.6468, 5.5) projected
  line L19 (45.6468, 5.5) -> (41.6468, 5.5) projected
  line L20 (41.6468, 5.5) -> (41.6468, 35.5) projected
  line L21 (41.6468, 35.5) -> (45.6468, 35.5) projected
  line L22 (21.6468, 35.5) -> (21.6468, 5.5) projected
  line L23 (21.6468, 5.5) -> (20.5, 5.5) projected
  line L24 (20.5, 35.5) -> (20.5, 5.5) projected
  line L25 (20.5, 35.5) -> (21.6468, 35.5) projected
  line L26 (113.45, 4) -> (60, 4) projected
  line L27 (60, 4) -> (60, 32.5785) projected
  line L28 (113.45, 32.5785) -> (113.45, 4) projected
  line L29 (21.6468, 5.5) -> (20.5, 5.5)
  line L30 (20.5, 5.5) -> (20.5, 35.5)
  line L31 (20.5, 35.5) -> (21.6468, 35.5)
  line L32 (21.6468, 35.5) -> (21.6468, 5.5)
  line L33 (60, 32.5785) -> (113.45, 32.5785) projected
  point P0 (124.7, 0)
  constraints: 8 end point, 2 parallel, 1 horizontal, 1 perpendicular
extrude "Extrusion22" add sketch "Sketch23" against normal up to surface (2.5 mm away) contours L22 L23 L24 L25
sketch "Sketch24" plane through (0, 0, 0) normal (1, 0, 0) x (0, 0, -1)
  line L0 (124.7, 30.6) -> (112.7, 30.6) projected
  line L1 (112.7, 30.6) -> (112.7, 40) projected
  line L2 (112.7, 40) -> (0, 40) projected
  line L3 (0, 0) -> (0, 40) projected
  line L4 (0, 0) -> (124.7, 0) projected
  line L5 (124.7, 0) -> (124.7, 30.6) projected
  line L6 (79.0532, 21.8) -> (79.0532, 35.5) projected
  line L7 (79.0532, 35.5) -> (83.0532, 35.5) projected
  line L8 (83.0532, 35.5) -> (83.0532, 21.8) projected
  line L9 (83.0532, 21.8) -> (79.0532, 21.8) projected
  line L10 (66, 17.8) -> (82, 17.8) projected
  line L11 (82, 17.8) -> (82, 5) projected
  line L12 (82, 5) -> (66, 5) projected
  line L13 (66, 5) -> (66, 17.8) projected
  line L14 (63.0532, 21.8) -> (63.0532, 35.5) projected
  line L15 (63.0532, 35.5) -> (67.0532, 35.5) projected
  line L16 (67.0532, 35.5) -> (67.0532, 21.8) projected
  line L17 (67.0532, 21.8) -> (63.0532, 21.8) projected
  line L18 (75.0532, 21.8) -> (71.0532, 21.8) projected
  line L19 (71.0532, 21.8) -> (71.0532, 35.5) projected
  line L20 (71.0532, 35.5) -> (75.0532, 35.5) projected
  line L21 (75.0532, 35.5) -> (75.0532, 21.8) projected
  line L22 (95.0532, 5.5) -> (95.0532, 35.5) projected
  line L23 (95.0532, 35.5) -> (99.0532, 35.5) projected
  line L24 (99.0532, 35.5) -> (99.0532, 5.5) projected
  line L25 (99.0532, 5.5) -> (95.0532, 5.5) projected
  line L26 (87.0532, 5.5) -> (87.0532, 35.5) projected
  line L27 (87.0532, 35.5) -> (91.0532, 35.5) projected
  line L28 (91.0532, 35.5) -> (91.0532, 5.5) projected
  line L29 (91.0532, 5.5) -> (87.0532, 5.5) projected
  line L30 (55.0532, 5.5) -> (55.0532, 35.5) projected
  line L31 (55.0532, 35.5) -> (59.0532, 35.5) projected
  line L32 (59.0532, 35.5) -> (59.0532, 5.5) projected
  line L33 (59.0532, 5.5) -> (55.0532, 5.5) projected
  line L34 (39.0532, 5.5) -> (39.0532, 35.5) projected
  line L35 (39.0532, 35.5) -> (43.0532, 35.5) projected
  line L36 (43.0532, 35.5) -> (43.0532, 5.5) projected
  line L37 (43.0532, 5.5) -> (39.0532, 5.5) projected
  line L38 (23.0532, 5.5) -> (23.0532, 35.5) projected
  line L39 (23.0532, 35.5) -> (27.0532, 35.5) projected
  line L40 (27.0532, 35.5) -> (27.0532, 5.5) projected
  line L41 (27.0532, 5.5) -> (23.0532, 5.5) projected
  line L42 (31.0532, 5.5) -> (31.0532, 35.5) projected
  line L43 (31.0532, 35.5) -> (35.0532, 35.5) projected
  line L44 (35.0532, 35.5) -> (35.0532, 5.5) projected
  line L45 (35.0532, 5.5) -> (31.0532, 5.5) projected
  line L46 (47.0532, 5.5) -> (47.0532, 35.5) projected
  line L47 (47.0532, 35.5) -> (51.0532, 35.5) projected
  line L48 (51.0532, 35.5) -> (51.0532, 5.5) projected
  line L49 (51.0532, 5.5) -> (47.0532, 5.5) projected
  line L50 (15.0532, 5.5) -> (15.0532, 35.5) projected
  line L51 (15.0532, 35.5) -> (19.0532, 35.5) projected
  line L52 (19.0532, 35.5) -> (19.0532, 5.5) projected
  line L53 (19.0532, 5.5) -> (15.0532, 5.5) projected
  line L54 (103.0532, 5.5) -> (103.0532, 35.5) projected
  line L55 (103.0532, 35.5) -> (107.0532, 35.5) projected
  line L56 (107.0532, 35.5) -> (107.0532, 5.5) projected
  line L57 (107.0532, 5.5) -> (103.0532, 5.5) projected
  line L58 (0, 0) -> (-40, 0)
  line L59 (-40, 0) -> (-40, 40)
  line L60 (-40, 40) -> (0, 40)
  line L61 (0, 40) -> (0, 0)
  circle A0 centre (-30, 30) radius 2.6
  circle A1 centre (-10, 30) radius 2.6
  circle A2 centre (-10, 10) radius 2.6
  circle A3 centre (-30, 10) radius 2.6
  dimension "d170" = 40
  dimension "d171" = 20
  dimension "d172" = 20
  dimension "d173" = 20
  dimension "d174" = 20
  dimension "d175" = 10
  dimension "d176" = 10
  dimension "d177" = 5.2
  dimension "d178" = 5.2
  dimension "d179" = 5.2
  dimension "d180" = 5.2
  constraints: 8 end point, 4 centre point, 4 coincident, 2 parallel, 1 horizontal, 1 perpendicular
  measures "d170" distance of L59.end L60.end
  measures "d171" distance of point (-10, 30) point (-30, 30)
  measures "d172" distance of point (-30, 30) point (-30, 10)
  measures "d173" distance of point (-10, 10) point (-30, 10)
  measures "d174" distance of point (-10, 30) point (-10, 10)
  measures "d175" distance from line of L58 point (-30, 10)
  measures "d176" distance from line of L59 point (-30, 10)
  measures "d177" diameter of A0
  measures "d178" diameter of A1
  measures "d179" diameter of A2
  measures "d180" diameter of A3
extrude "Extrusion23" add sketch "Sketch24" along normal blind 2.5
sketch "Sketch25" plane through (2.5, 0, 0) normal (1, 0, 0) x (0, 0, -1)
  line L0 (82, 17.8) -> (82, 5) projected
  line L1 (82, 5) -> (66, 5) projected
  line L2 (66, 5) -> (66, 17.8) projected
  line L3 (66, 17.8) -> (82, 17.8) projected
  line L4 (103.0532, 35.5) -> (107.0532, 35.5) projected
  line L5 (107.0532, 35.5) -> (107.0532, 5.5) projected
  line L6 (107.0532, 5.5) -> (103.0532, 5.5) projected
  line L7 (103.0532, 5.5) -> (103.0532, 35.5) projected
  line L8 (15.0532, 35.5) -> (19.0532, 35.5) projected
  line L9 (19.0532, 35.5) -> (19.0532, 5.5) projected
  line L10 (19.0532, 5.5) -> (15.0532, 5.5) projected
  line L11 (15.0532, 5.5) -> (15.0532, 35.5) projected
  line L12 (47.0532, 35.5) -> (51.0532, 35.5) projected
  line L13 (51.0532, 35.5) -> (51.0532, 5.5) projected
  line L14 (51.0532, 5.5) -> (47.0532, 5.5) projected
  line L15 (47.0532, 5.5) -> (47.0532, 35.5) projected
  line L16 (31.0532, 35.5) -> (35.0532, 35.5) projected
  line L17 (35.0532, 35.5) -> (35.0532, 5.5) projected
  line L18 (35.0532, 5.5) -> (31.0532, 5.5) projected
  line L19 (31.0532, 5.5) -> (31.0532, 35.5) projected
  line L20 (23.0532, 35.5) -> (27.0532, 35.5) projected
  line L21 (27.0532, 35.5) -> (27.0532, 5.5) projected
  line L22 (27.0532, 5.5) -> (23.0532, 5.5) projected
  line L23 (23.0532, 5.5) -> (23.0532, 35.5) projected
  line L24 (39.0532, 35.5) -> (43.0532, 35.5) projected
  line L25 (43.0532, 35.5) -> (43.0532, 5.5) projected
  line L26 (43.0532, 5.5) -> (39.0532, 5.5) projected
  line L27 (39.0532, 5.5) -> (39.0532, 35.5) projected
  line L28 (55.0532, 35.5) -> (59.0532, 35.5) projected
  line L29 (59.0532, 35.5) -> (59.0532, 5.5) projected
  line L30 (59.0532, 5.5) -> (55.0532, 5.5) projected
  line L31 (55.0532, 5.5) -> (55.0532, 35.5) projected
  line L32 (87.0532, 35.5) -> (91.0532, 35.5) projected
  line L33 (91.0532, 35.5) -> (91.0532, 5.5) projected
  line L34 (91.0532, 5.5) -> (87.0532, 5.5) projected
  line L35 (87.0532, 5.5) -> (87.0532, 35.5) projected
  line L36 (95.0532, 35.5) -> (99.0532, 35.5) projected
  line L37 (99.0532, 35.5) -> (99.0532, 5.5) projected
  line L38 (99.0532, 5.5) -> (95.0532, 5.5) projected
  line L39 (95.0532, 5.5) -> (95.0532, 35.5) projected
  line L40 (71.0532, 21.8) -> (71.0532, 35.5) projected
  line L41 (71.0532, 35.5) -> (75.0532, 35.5) projected
  line L42 (75.0532, 35.5) -> (75.0532, 21.8) projected
  line L43 (75.0532, 21.8) -> (71.0532, 21.8) projected
  line L44 (63.0532, 35.5) -> (67.0532, 35.5) projected
  line L45 (67.0532, 35.5) -> (67.0532, 21.8) projected
  line L46 (67.0532, 21.8) -> (63.0532, 21.8) projected
  line L47 (63.0532, 21.8) -> (63.0532, 35.5) projected
  line L48 (79.0532, 35.5) -> (83.0532, 35.5) projected
  line L49 (83.0532, 35.5) -> (83.0532, 21.8) projected
  line L50 (83.0532, 21.8) -> (79.0532, 21.8) projected
  line L51 (79.0532, 21.8) -> (79.0532, 35.5) projected
  circle A0 centre (-30, 10) radius 2.6 projected
  circle A1 centre (-10, 10) radius 2.6 projected
  circle A2 centre (-10, 30) radius 2.6 projected
  circle A3 centre (-30, 30) radius 2.6 projected
  line L52 (112.7, 40) -> (-40, 40) projected
  line L53 (-40, 40) -> (-40, 0) projected
  line L54 (-40, 0) -> (124.7, 0) projected
  line L55 (124.7, 0) -> (124.7, 30.6) projected
  line L56 (124.7, 30.6) -> (112.7, 30.6) projected
  line L57 (112.7, 30.6) -> (112.7, 40) projected
  line L58 (107.0532, 5.5) -> (103.0532, 5.5)
  line L59 (103.0532, 5.5) -> (103.0532, 35.5)
  line L60 (103.0532, 35.5) -> (107.0532, 35.5)
  line L61 (107.0532, 35.5) -> (107.0532, 5.5)
  point P0 (0, 0)
  constraints: 8 end point, 2 parallel, 1 horizontal, 1 perpendicular
extrude "Extrusion24" add sketch "Sketch25" against normal blind 5 contours L4 L5 L6 L7
sketch "Sketch26" plane through (-2.5, 2, -104.2) normal (-1, 0, 0) x (0, 0, 1)
  line L0 (9.1468, 33.5) -> (9.1468, 3.5) projected
  line L1 (9.1468, 3.5) -> (5.1468, 3.5) projected
  line L2 (5.1468, 3.5) -> (5.1468, 33.5) projected
  line L3 (5.1468, 33.5) -> (9.1468, 33.5) projected
  line L4 (17.1468, 33.5) -> (17.1468, 3.5) projected
  line L5 (17.1468, 3.5) -> (13.1468, 3.5) projected
  line L6 (13.1468, 3.5) -> (13.1468, 33.5) projected
  line L7 (13.1468, 33.5) -> (17.1468, 33.5) projected
  line L8 (49.1468, 33.5) -> (49.1468, 3.5) projected
  line L9 (49.1468, 3.5) -> (45.1468, 3.5) projected
  line L10 (45.1468, 3.5) -> (45.1468, 33.5) projected
  line L11 (45.1468, 33.5) -> (49.1468, 33.5) projected
  line L12 (65.1468, 33.5) -> (65.1468, 3.5) projected
  line L13 (65.1468, 3.5) -> (61.1468, 3.5) projected
  line L14 (61.1468, 3.5) -> (61.1468, 33.5) projected
  line L15 (61.1468, 33.5) -> (65.1468, 33.5) projected
  line L16 (81.1468, 33.5) -> (81.1468, 3.5) projected
  line L17 (81.1468, 3.5) -> (77.1468, 3.5) projected
  line L18 (77.1468, 3.5) -> (77.1468, 33.5) projected
  line L19 (77.1468, 33.5) -> (81.1468, 33.5) projected
  line L20 (73.1468, 33.5) -> (73.1468, 3.5) projected
  line L21 (73.1468, 3.5) -> (69.1468, 3.5) projected
  line L22 (69.1468, 3.5) -> (69.1468, 33.5) projected
  line L23 (69.1468, 33.5) -> (73.1468, 33.5) projected
  line L24 (57.1468, 33.5) -> (57.1468, 3.5) projected
  line L25 (57.1468, 3.5) -> (53.1468, 3.5) projected
  line L26 (53.1468, 3.5) -> (53.1468, 33.5) projected
  line L27 (53.1468, 33.5) -> (57.1468, 33.5) projected
  line L28 (89.1468, 33.5) -> (89.1468, 3.5) projected
  line L29 (89.1468, 3.5) -> (85.1468, 3.5) projected
  line L30 (85.1468, 3.5) -> (85.1468, 33.5) projected
  line L31 (85.1468, 33.5) -> (89.1468, 33.5) projected
  line L32 (92.95, 38) -> (0, 38) projected
  line L33 (0, 33.5) -> (0, 38) projected
  line L34 (-2.8532, 33.5) -> (0, 33.5) projected
  line L35 (-2.8532, 3.5) -> (-2.8532, 33.5) projected
  line L36 (0, 3.5) -> (-2.8532, 3.5) projected
  line L37 (0, 0) -> (0, 3.5) projected
  line L38 (0, 0) -> (92.95, 0) projected
  line L39 (92.95, 38) -> (92.95, 0) projected
  line L40 (41.1468, 19.8) -> (37.1468, 19.8) projected
  line L41 (37.1468, 19.8) -> (37.1468, 33.5) projected
  line L42 (37.1468, 33.5) -> (41.1468, 33.5) projected
  line L43 (41.1468, 33.5) -> (41.1468, 19.8) projected
  line L44 (25.1468, 19.8) -> (21.1468, 19.8) projected
  line L45 (21.1468, 19.8) -> (21.1468, 33.5) projected
  line L46 (21.1468, 33.5) -> (25.1468, 33.5) projected
  line L47 (25.1468, 33.5) -> (25.1468, 19.8) projected
  line L48 (29.1468, 19.8) -> (29.1468, 33.5) projected
  line L49 (29.1468, 33.5) -> (33.1468, 33.5) projected
  line L50 (33.1468, 33.5) -> (33.1468, 19.8) projected
  line L51 (33.1468, 19.8) -> (29.1468, 19.8) projected
  line L52 (22.2, 15.8) -> (38.2, 15.8) projected
  line L53 (38.2, 15.8) -> (38.2, 3) projected
  line L54 (38.2, 3) -> (22.2, 3) projected
  line L55 (22.2, 3) -> (22.2, 15.8) projected
  line L56 (0, 3.5) -> (-2.8532, 3.5) projected
  line L57 (0, 33.5) -> (-2.8532, 33.5)
  line L58 (-2.8532, 33.5) -> (-2.8532, 3.5)
  line L59 (-2.8532, 3.5) -> (0, 3.5)
  line L60 (0, 3.5) -> (0, 33.5)
  point P0 (104.2, -2)
  constraints: 8 end point, 2 parallel, 1 horizontal, 1 perpendicular
extrude "Extrusion25" add sketch "Sketch26" along normal up to surface (8.5 mm away) contours L60 L36 L35 L34
sketch "Sketch27" plane through (0, 40, 0) normal (0, 1, 0) x (1, 0, 0)
  line L0 (-113, 112.7) -> (-124, 112.7) projected
  line L1 (-124, 0) -> (-124, 112.7) projected
  line L2 (0, 0) -> (-124, 0) projected
  line L3 (0, 0) -> (0, -40) projected
  line L4 (0, -40) -> (2.5, -40) projected
  line L5 (2.5, 112.7) -> (2.5, -40) projected
  line L6 (2.5, 112.7) -> (-11, 112.7) projected
  line L7 (-11, 104.2) -> (-11, 112.7) projected
  line L8 (-2.5, 104.2) -> (-11, 104.2) projected
  line L9 (-2.5, 11.25) -> (-2.5, 104.2) projected
  line L10 (-11, 11.25) -> (-2.5, 11.25) projected
  line L11 (-11, 2.5) -> (-11, 11.25) projected
  line L12 (-113, 2.5) -> (-11, 2.5) projected
  line L13 (-113, 11.25) -> (-113, 2.5) projected
  line L14 (-121.5, 11.25) -> (-113, 11.25) projected
  line L15 (-121.5, 104.2) -> (-121.5, 11.25) projected
  line L16 (-113, 104.2) -> (-121.5, 104.2) projected
  line L17 (-113, 112.7) -> (-113, 104.2) projected
  circle A0 centre (-117.375, 108.45) radius 1.35 projected
  circle A1 centre (-6.625, 108.45) radius 1.35 projected
  circle A2 centre (-6.625, 6.875) radius 1.35 projected
  circle A3 centre (-117.375, 6.875) radius 1.35 projected
  line L18 (-121.5, 112.7) -> (-2.5, 112.7)
  line L19 (-2.5, 112.7) -> (-2.5, 2.5)
  line L20 (-2.5, 2.5) -> (-121.5, 2.5)
  line L21 (-121.5, 2.5) -> (-121.5, 112.7)
  constraints: 8 end point, 2 parallel, 1 horizontal, 1 perpendicular, 1 point on line
extrude "Extrusion26" cut sketch "Sketch27" against normal blind 2.5 contours L17 L16 L21 L0 | L18 L7 L8 L9 L10 L11 L12 L13 L14 L15 L16 L17 | L6 L19 L8 L7 | L14 L13 L20 L21 | L19 L20 L11 L10
fillet "Fillet2" radius 3 3 edges at (-113, 19.75, -11.25) (-11, 19.75, -11.25) (-11, 19.75, -104.2)